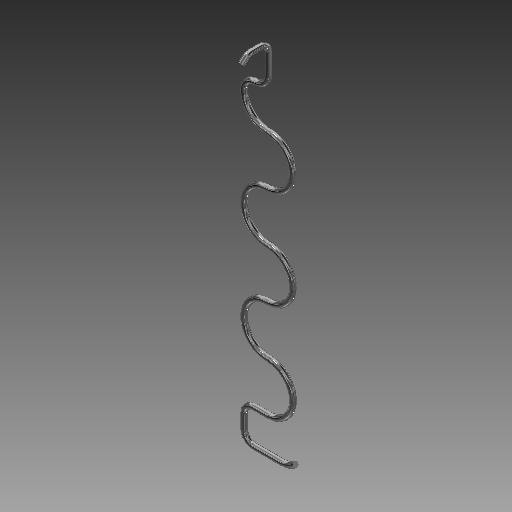
# Autodesk Inventor part: 314-12
Saved by Autodesk Inventor 2019 (Build 230136000, 136)
## iProperties
Company: Autodesk Inc.
Created: 2007-11-01
Part Number: 314-12
Document SubType Name: Modeling
Designer: Autodesk Inc.
Density: 8 g/cm^3
Mass: 45.5929 g
Surface Area: 57.2425 cm^2
Volume: 5.69911 cm^3
Material: Stainless Steel
Description: SPRING WIRE
Appearance: Steel - Polished
Component Category: Lower Component
Author: Inventor
Autodesk Inventor part; units mm, degrees
ref_plane "YZ Plane" through (0, 0, 0) normal (1, 0, 0) x (0, 1, 0)
ref_plane "XZ Plane" through (0, 0, 0) normal (0, 1, 0) x (-1, 0, 0)
sketch "Sketch1" plane through (0, 0, 0) normal (0, 0, 1) x (1, 0, 0)
  line L0 (10, 0) -> (-10, 0)
  line L1 (-18, 8) -> (-18, 17)
  line L2 (-10, 25) -> (0, 25)
  line L3 (18.6036, 2.7127) -> (19.7295, 3.501)
  arc A0 (-10, 25) -> (-18, 17) centre (-10, 17) ccw
  arc A1 (-18, 8) -> (-10, 0) centre (-10, 8) ccw
  arc A2 (10, 0) -> (18.6036, 2.7127) centre (10, 15) ccw
  line L4 (0, 241) -> (0, 279.2364) construction
  arc A3 (0, 25) -> (0, 61) centre (0, 43) ccw
  arc A4 (0, 97) -> (0, 61) centre (0, 79) ccw
  arc A5 (0, 169) -> (0, 133) centre (0, 151) ccw
  arc A6 (-18, 223) -> (0, 205) centre (0, 223) ccw
  arc A7 (-9, 232) -> (-18, 223) centre (-9, 223) ccw
  line L5 (0, 223) -> (-9, 223) construction
  line L6 (0, 241) -> (0, 246.7859)
  line L7 (0, 97) -> (0, 133) construction
  line L8 (0, 169) -> (0, 205) construction
  arc A8 (0, 97) -> (0, 133) centre (0, 115) ccw
  arc A9 (0, 169) -> (0, 205) centre (0, 187) ccw
  arc A10 (-9, 232) -> (0, 241) centre (-9, 241) ccw
  point P0 (0, 0)
  point P1 (14.7295, 0)
  point P2 (-18, 0)
  point P3 (-18, 25)
  point P4 (0, 0)
  dimension "d1" = 5
  dimension "d2" = 35
  dimension "d3" = 25
  dimension "d5" = 8
  dimension "d6" = 18
  dimension "d7" = 15
  dimension "d10" = 36
  dimension "d11" = 36
  dimension "d13" = 36
  dimension "d17" = 18
  dimension "d18" = 9
  dimension "d19" = 151
  dimension "d20" = 223
  dimension "d21" = 9
  dimension "d22" = 18
  dimension "d23" = 9
  constraints: 22 point on circle, 16 end point, 11 centre point, 9 tangent, 6 point on line, 3 midpoint, 2 collinear, 2 horizontal, 2 parallel, 1 coincident, 1 equal radius, 1 perpendicular, 14 other
  measures "d1" horizontal distance of L3.end point (14.729, 0)
  measures "d2" angle of L0 L3
  measures "d3" distance of point (-18, 0) point (-18, 25)
  measures "d5" radius of A0
  measures "d6" distance from line of point (0, 0) L1
  measures "d7" radius of A2
  measures "d10" diameter of A3
  measures "d11" diameter of A4
  measures "d13" diameter of A5
  measures "d17" radius of A6
  measures "d18" radius of A7
  measures "d19" distance from line of A5.centre L0
  measures "d20" distance of L5.start point (0, 0)
  measures "d22" vertical distance of L5.start A10.centre
  measures "d23" radius of A10
ref_plane "Work Plane1" through (19.7295, 3.501, 0) normal (0.8192, 0.5736, 0) x (-0.5736, 0.8192, 0)
sketch "Sketch2" plane through (19.7295, 3.501, 0) normal (0.8192, 0.5736, 0) x (-0.5736, 0.8192, 0)
  circle A0 centre (0, 0) radius 2
  point P0 (8.4485, 0)
  dimension "d8" = 4
  constraints: 1 centre point
  measures "d8" diameter of A0
sweep "Sweep2" add profiles "Sketch2" path "Sketch1"
sketch "Sketch3" plane through (0, 0, 0) normal (1, 0, 0) x (0, 1, 0)
  line L0 (246.7859, 2) -> (246.7859, -2) projected
  line L1 (246.7859, 0) -> (255.7859, 0)
  line L2 (261.7859, 6) -> (261.7859, 12.8162)
  line L3 (260.3822, 16.6729) -> (257.5904, 20)
  arc A0 (255.7859, 0) -> (261.7859, 6) centre (255.7859, 6) ccw
  arc A1 (261.7859, 12.8162) -> (260.3822, 16.6729) centre (255.7859, 12.8162) ccw
  point P0 (0, 0)
  point P1 (261.7859, 0)
  point P2 (261.7859, 15)
  dimension "d25" = 15
  dimension "d26" = 15
  dimension "d27" = 40
  dimension "d28" = 5
  dimension "d29" = 6
  constraints: 6 end point, 4 point on circle, 4 point on line, 4 tangent, 2 centre point, 2 perpendicular, 1 equal radius, 1 midpoint
  measures "d25" distance of L1.start point (261.786, 0)
  measures "d26" distance of point (261.786, 0) point (261.786, 15)
  measures "d27" angle of L2 L3
  measures "d28" vertical distance of point (261.786, 15) L3.end
  measures "d29" radius of A0
sketch "Sketch4" plane through (0, 246.7859, 0) normal (0, 1, 0) x (1, 0, 0)
  circle A0 centre (0, 0) radius 2 projected
sweep "Sweep3" add profiles "Sketch4" path "Sketch3" path curves L1 A0 L2 A1 L3
equation "\"d11\" = d10"
equation "\"d13\" = d10"
equation "\"d15\" = d10"
body "Solid1"
